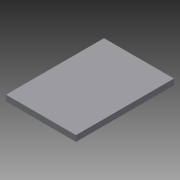
# Autodesk Inventor part: CURM_CaterpillarBody
Saved by Autodesk Inventor 2015 (Build 190159000, 159)
## iProperties
Created: 2015-02-11
Part Number: CURM_CaterpillarBody
Material: Generic
Document SubType Name: Modeling
Designer: Judson
Density: 1 g/cm^3
Appearance: Default
Author: Judson
Autodesk Inventor part; units mm, degrees
ref_plane "YZ Plane" through (0, 0, 0) normal (1, 0, 0) x (0, 1, 0)
ref_plane "XZ Plane" through (0, 0, 0) normal (0, 1, 0) x (-1, 0, 0)
ref_plane "XY Plane" through (0, 0, 0) normal (0, 0, 1) x (1, 0, 0)
sketch "Sketch1" plane through (0, 0, 0) normal (0, 1, 0) x (-1, 0, 0)
  line L0 (19.05, -26.67) -> (-19.05, -26.67)
  line L1 (-19.05, -26.67) -> (-19.05, 26.67)
  line L2 (-19.05, 26.67) -> (19.05, 26.67)
  line L3 (19.05, 26.67) -> (19.05, -26.67)
  point P0 (0, 0)
  dimension "d0" = 53.34
  dimension "d1" = 19.05
  dimension "d2" = 38.1
  dimension "d3" = 26.67
  constraints: 8 end point, 2 parallel, 1 horizontal, 1 perpendicular
  measures "d0" distance of L0.end L1.end
  measures "d1" distance from line of L1 point (0, 0)
  measures "d2" distance of L1.end L2.end
  measures "d3" distance from line of point (0, 0) L0
extrude "bottom panel" add sketch "Sketch1" along normal blind 3.175
body "Solid1"
